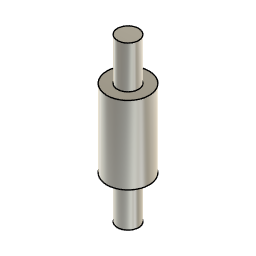
MM_FRAME_SPACER_M6 (Autodesk Fusion 360 design; units mm, degrees)
Autodesk Fusion 360 part; units mm, degrees
sketch "Esquisse1" plane through (0, 0, 0) normal (0, 0, 1) x (1, 0, 0)
  circle A0 centre (0, 0) radius 6
  dimension "d1" = 12
  constraint coincident A0.centre origin
  measures "d1" diameter of A0
extrude "Extrusion1" add sketch "Esquisse1" along normal blind 22
sketch "Esquisse2" plane through (0, 0, 22) normal (0, 0, 1) x (-1, 0, 0)
  circle A0 centre (0, 0) radius 6
  circle A1 centre (0, 0) radius 3
  dimension "d4" = 6
  constraint concentric A0 A1
  measures "d4" diameter of A1
extrude "Extrusion2" add sketch "Esquisse2" along normal blind 12 contours A1
sketch "Esquisse3" plane through (0, 0, 0) normal (0, 0, -1) x (1, 0, 0)
  circle A0 centre (0, 0) radius 6
  circle A1 centre (0, 0) radius 3
  dimension "d7" = 6
  constraint concentric A0 A1
  measures "d7" diameter of A1
extrude "Extrusion3" add sketch "Esquisse3" along normal blind 12 contours A1
